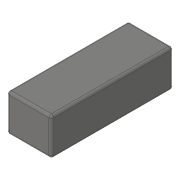
# Autodesk Inventor part: 850mah
Saved by Autodesk Inventor 2019 (Build 230136000, 136)
## iProperties
Created: 2022-04-02
Part Number: 850mah
Material: Battery
Document SubType Name: Modeling
Designer: solyo
Density: 2.10367 g/cm^3
Appearance: Battery
Mass: 27.6863 g
Surface Area: 36.3209 cm^2
Volume: 13.1609 cm^3
Author: solyo
Autodesk Inventor part; units mm, degrees
ref_plane "YZ Plane" through (0, 0, 0) normal (1, 0, 0) x (0, 1, 0)
ref_plane "XZ Plane" through (0, 0, 0) normal (0, 1, 0) x (-1, 0, 0)
ref_plane "XY Plane" through (0, 0, 0) normal (0, 0, 1) x (1, 0, 0)
sketch "Sketch1" plane through (0, 0, 0) normal (0, 0, 1) x (1, 0, 0)
  line L0 (9, -7.5) -> (-9, -7.5)
  line L1 (-9, -7.5) -> (-9, 7.5)
  line L2 (-9, 7.5) -> (9, 7.5)
  line L3 (9, 7.5) -> (9, -7.5)
  line L4 (9, -7.5) -> (-9, 7.5) construction
  line L5 (-9, -7.5) -> (9, 7.5) construction
  point P0 (0, 0)
  dimension "d0" = 18
  dimension "d1" = 15
  constraints: 12 end point, 2 midpoint, 2 parallel, 1 horizontal, 1 perpendicular
  measures "d0" distance of L1.end L2.end
  measures "d1" distance of L0.end L1.end
extrude "Extrusion1" add sketch "Sketch1" along normal mid plane 49
fillet "Fillet1" radius 1 12 edges at (0, 7.5, 24.5) (9, 0, 24.5) (-9, 0, 24.5) (0, -7.5, 24.5) (9, -7.5, 0) (9, 7.5, 0) (-9, 7.5, 0) (-9, -7.5, 0) (0, 7.5, -24.5) (9, 0, -24.5) (-9, 0, -24.5) (0, -7.5, -24.5)
body "Solid1"
